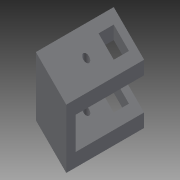
# Autodesk Inventor part: gimbal_stick_fixation_big
Saved by Autodesk Inventor 2015 SP1 (Build 190203100, 203)
## iProperties
Created: 2015-07-15
Part Number: gimbal_stick_fixation_big
Material: Generic
Document SubType Name: Modeling
Designer: Alexandre Cherpillod
Density: 1 g/cm^3
Appearance: Default
Author: Alexandre Cherpillod
Autodesk Inventor part; units mm, degrees
ref_plane "YZ Plane" through (0, 0, 0) normal (1, 0, 0) x (0, 1, 0)
ref_plane "XZ Plane" through (0, 0, 0) normal (0, 1, 0) x (-1, 0, 0)
ref_plane "XY Plane" through (0, 0, 0) normal (0, 0, 1) x (1, 0, 0)
sketch "Sketch2" plane through (0, 0, 0) normal (0, 1, 0) x (-1, 0, 0)
  line L0 (0, 0) -> (15.6172, 15.6172) construction
  line L1 (0, 0) -> (0, -11.6637) construction
  line L2 (-18.4102, -9.9249) -> (9.458, 17.9433) construction
  line L3 (0, 0) -> (8, 8)
  line L4 (8, 4.4645) -> (8, 4.4645)
  line L5 (8, 8) -> (8, 4.4645)
  line L6 (0, 0) -> (0, -3.5355)
  line L7 (0, 8.4853) -> (0, 12.0208)
  line L8 (0, 12.0208) -> (8, 20.0208)
  line L9 (8, 20.0208) -> (8, 16.4853)
  line L10 (0, 8.4853) -> (8, 16.4853)
  line L11 (8, 4.4645) -> (0, -3.5355)
  point P0 (-12.2426, -3.7574)
  dimension "d0" = 135
  dimension "d1" = 6
  dimension "d2" = 2.5
  dimension "d4" = 8
  constraints: 24 end point, 6 point on line, 4 collinear, 3 parallel, 3 vertical
  measures "d0" angle of L0 L1
  measures "d1" distance between parallel lines of L0 L2
  measures "d2" distance between parallel lines of L0 L4
  measures "d4" horizontal distance of L4.end L6.end
extrude "Extrusion1" add sketch "Sketch2" along normal blind 18
sketch "Sketch3" plane through (0, 0, 0) normal (0, -1, 0) x (1, 0, 0)
  line L0 (-8, 20.0208) -> (0, 12.0208) projected
  line L1 (-8, 4.4645) -> (0, -3.5355) projected
  line L2 (-8, 8) -> (-8, 4.4645) projected
  line L3 (0, 26.3321) -> (0, -17.8468) projected
  line L4 (-8, 16.4853) -> (-8, 20.0208) projected
  line L5 (0, 12.0208) -> (0, -3.5355)
  line L6 (-8, 4.4645) -> (-8, 20.0208)
  line L7 (-8, 20.0208) -> (0, 12.0208)
  line L8 (0, -3.5355) -> (-8, 4.4645)
  point P0 (0, 0)
  constraints: 8 end point, 2 collinear, 1 vertical
extrude "Extrusion2" add sketch "Sketch3" along normal blind 2.5
sketch "Sketch4" plane through (0, 0, 0) normal (0, 0, 1) x (1, 0, 0)
  line L0 (-8, 18) -> (0, 18) projected
  line L1 (-2, 16) -> (-6, 16)
  line L2 (-6, 16) -> (-6, 12)
  line L3 (-6, 12) -> (-2, 12)
  line L4 (-2, 12) -> (-2, 16)
  line L5 (-4, 18) -> (-4, 0)
  line L6 (0, 0) -> (-8, 0) projected
  point P0 (-4, 16)
  dimension "d9" = 4
  dimension "d10" = 4
  dimension "d14" = 12
  constraints: 10 end point, 2 midpoint, 2 parallel, 1 horizontal, 1 perpendicular, 1 point on line, 1 vertical
  measures "d9" distance of L1.start L1.end
  measures "d10" distance of L1.end L2.end
  measures "d14" distance between parallel lines of L6 L3
extrude "Extrusion3" cut sketch "Sketch4" along normal through all both and the other way through all
sketch "Sketch6" plane through (0, 0, 0) normal (0, 0, 1) x (1, 0, 0)
  line L0 (-2, 12) -> (-6, 12) projected
  line L1 (-4, 12) -> (-4, 2.9314) construction
  circle A0 centre (-4, 6.75) radius 0.75
  line L2 (0, 0) -> (-8, 0) projected
  dimension "d20" = 1.5
  dimension "d21" = 6
  constraints: 2 end point, 1 centre point, 1 midpoint, 1 point on line, 1 vertical
  measures "d20" diameter of A0
  measures "d21" distance edge to line of A0 L2
extrude "Extrusion5" cut sketch "Sketch6" along normal through all both and the other way through all
body "Solid1"
